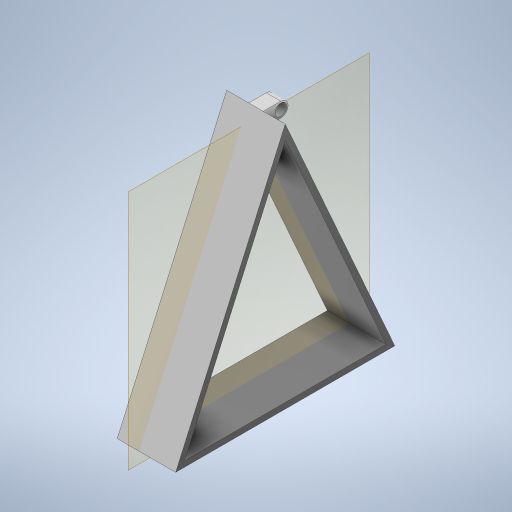
# Autodesk Inventor part: SensorArm
Saved by Autodesk Inventor 2023 (Build 270158000, 158)
## iProperties
Created: 2024-01-25
Part Number: SensorArm
Material: Generisch
Document SubType Name: Modeling
Designer: phili
Density: 1 g/cm^3
Appearance: Vorgabe
Author: phili
Autodesk Inventor part; units mm, degrees
ref_plane "XZ Plane" through (0, 0, 0) normal (0, 1, 0) x (-1, 0, 0)
ref_plane "XY Plane" through (0, 0, 0) normal (0, 0, 1) x (1, 0, 0)
sketch "Skizze1" plane through (0, 0, 0) normal (1, 0, 0) x (0, 1, 0)
  line L0 (0, 75) -> (0, -75)
  line L1 (0, 75) -> (150, 75) construction
  line L2 (0, 75) -> (169.007, 0)
  line L3 (169.007, 0) -> (0, -75)
  point P0 (0, 0)
  point P1 (0, 0)
  dimension "d0" = 150
  dimension "d1" = 90
  dimension "d2" = 75
  dimension "d3" = 169.007
  constraints: 8 end point, 1 horizontal, 1 midpoint, 1 perpendicular, 1 vertical
  measures "d0" distance of L0.start L0.end
  measures "d1" angle of L0 L1
  measures "d2" distance of L0.start point (0, 0)
  measures "d3" distance of point (0, 0) L2.end
extrude "Extrusion1" add sketch "Skizze1" along normal blind 40
shell "Wandung1" thickness 4 removed faces 2 at (40, 56.3357, 0) at (0, 56.3357, 0)
ref_plane "Arbeitsebene3" through (15, 0, 0) normal (1, 0, 0) x (0, 1, 0)
sketch "Skizze7" plane through (15, 0, 0) normal (1, 0, 0) x (0, 1, 0)
  line L0 (0, -75) -> (169.007, 0) projected
  line L1 (169.007, 0) -> (169.007, -17)
  line L2 (169.007, -17) -> (159.007, -17)
  line L3 (159.007, -17) -> (159.007, -4.4377)
  point P0 (0, 0)
  dimension "d24" = 17
  dimension "d25" = 10
  constraints: 6 end point, 2 perpendicular, 1 point on line, 1 vertical
  measures "d24" distance of L0.end L1.end
  measures "d25" distance of L1.end L2.end
extrude "Extrusion6" add sketch "Skizze7" along normal blind 10
fillet "Rundung1" radius 5 2 edges at (20, 159.007, -17) (20, 169.007, -17)
sketch "Skizze8" plane through (25, 0, 0) normal (1, 0, 0) x (0, 0, -1)
  arc A0 (12, 159.007) -> (12, 169.007) centre (12, 164.007) ccw projected
  circle A1 centre (12, 164.007) radius 4
  point P0 (0, 0)
  dimension "d29" = 8
  constraints: 1 centre point, 1 coincident
  measures "d29" diameter of A1
extrude "Extrusion7" cut sketch "Skizze8" against normal through all
